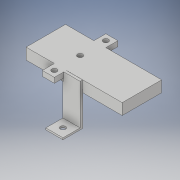
# Autodesk Inventor part: New poe ethernet splitter holder
Saved by Autodesk Inventor 2018 (Build 220112000, 112)
## iProperties
Created: 2019-11-08
Part Number: New poe ethernet splitter holder
Material: Generic
Document SubType Name: Modeling
Designer: Jacob
Density: 1 g/cm^3
Appearance: Default
Author: Jacob
Autodesk Inventor part; units mm, degrees
ref_plane "YZ Plane" through (0, 0, 0) normal (1, 0, 0) x (0, 1, 0)
ref_plane "XZ Plane" through (0, 0, 0) normal (0, 1, 0) x (-1, 0, 0)
ref_plane "XY Plane" through (0, 0, 0) normal (0, 0, 1) x (1, 0, 0)
sketch "Sketch1" plane through (0, 0, 0) normal (0, 1, 0) x (-1, 0, 0)
  line L0 (5, -5) -> (-5, -5)
  line L1 (-5, -5) -> (-5, 5)
  line L2 (-5, 5) -> (5, 5)
  line L3 (5, 5) -> (5, -5)
  line L4 (5, -5) -> (-5, 5) construction
  line L5 (-5, -5) -> (5, 5) construction
  circle A0 centre (0, 0) radius 1.5
  dimension "d0" = 10
  dimension "d1" = 10
  dimension "d2" = 3
  constraints: 12 end point, 2 midpoint, 2 parallel, 1 centre point, 1 coincident, 1 horizontal, 1 perpendicular
  measures "d0" distance of L0.start L0.end
  measures "d1" distance of L0.end L1.end
  measures "d2" diameter of A0
extrude "Extrusion1" add sketch "Sketch1" along normal blind 1
sketch "Sketch2" plane through (0, 1, 0) normal (0, 1, 0) x (1, 0, 0)
  line L0 (5, 5) -> (-5, 5) projected
  line L1 (-5, 5) -> (5, 5)
  line L2 (5, 5) -> (5, 6.5)
  line L3 (5, 6.5) -> (-5, 6.5)
  line L4 (-5, 6.5) -> (-5, 5)
  point P0 (0, 0)
  dimension "d5" = 1.5
  constraints: 8 end point, 2 parallel, 1 horizontal, 1 perpendicular
  measures "d5" distance of L1.end L2.end
extrude "Extrusion2" add sketch "Sketch2" against normal blind 1
sketch "Sketch3" plane through (0, 1, 0) normal (0, 1, 0) x (1, 0, 0)
  line L0 (-5, 6.5) -> (-5, -5) projected
  line L1 (5, -5) -> (5, 6.5) projected
  line L2 (-5, 6.5) -> (5, 6.5)
  line L3 (5, 6.5) -> (5, 5)
  line L4 (5, 5) -> (-5, 5)
  line L5 (-5, 5) -> (-5, 6.5)
  point P0 (0, 0)
  dimension "d8" = 1.5
  constraints: 8 end point, 2 parallel, 1 horizontal, 1 perpendicular, 1 point on line
  measures "d8" distance between parallel lines of L2 L4
extrude "Extrusion3" add sketch "Sketch3" along normal blind 17
sketch "Sketch4" plane through (0, 18, 0) normal (0, 1, 0) x (1, 0, 0)
  line L0 (-5, 5) -> (5, 5) projected
  line L1 (5, 6.5) -> (-5, 6.5) projected
  line L2 (-5, 6.5) -> (-5, 5) projected
  line L3 (5, 5) -> (5, 6.5) projected
  point P0 (0, 0)
extrude "Extrusion4" add sketch "Sketch4" along normal blind 1.5
sketch "Sketch5" plane through (5, 0, -6.5) normal (0, 0, -1) x (-1, 0, 0)
  line L0 (5, 0) -> (5, 19.5) construction
  line L1 (0, 19.5) -> (10, 19.5) projected
  line L2 (-23, 19.5) -> (33, 19.5)
  line L3 (33, 19.5) -> (33, 18)
  line L4 (33, 18) -> (-23, 18)
  line L5 (-23, 18) -> (-23, 19.5)
  line L6 (-23, 19.5) -> (33, 18) construction
  line L7 (33, 19.5) -> (-23, 18) construction
  point P0 (5, 18.75)
  dimension "d13" = 0
  dimension "d14" = 1.5
  dimension "d15" = 56
  constraints: 14 end point, 3 midpoint, 2 parallel, 1 horizontal, 1 perpendicular, 1 point on line
  measures "d13" distance between parallel lines of L1 L2
  measures "d14" distance of L4.end L2.start
  measures "d15" distance of L3.end L4.end
extrude "Extrusion5" add sketch "Sketch5" along normal blind 23
sketch "Sketch6" plane through (0, 19.5, 0) normal (0, 1, 0) x (1, 0, 0)
  line L0 (-28, 6.5) -> (-28, 29.5) projected
  line L1 (-28, 18) -> (28, 18) construction
  line L2 (28, 6.5) -> (28, 29.5) projected
  circle A0 centre (-8, 18) radius 1.5
  line L3 (-5, 6.5) -> (-28, 6.5) projected
  line L4 (-28, 29.5) -> (28, 29.5) projected
  line L5 (-5, 6.5) -> (5, 6.5) projected
  line L6 (28, 6.5) -> (5, 6.5) projected
  point P0 (0, 0)
  dimension "d18" = 20
  dimension "d19" = 3
  constraints: 2 end point, 2 midpoint, 1 centre point, 1 point on line
  measures "d18" distance from line of L0 A0.centre
  measures "d19" diameter of A0
extrude "Extrusion6" add sketch "Sketch6" along normal blind 5
sketch "Sketch8" plane through (0, 24.5, 0) normal (0, 1, 0) x (1, 0, 0)
  line L0 (-28, 6.5) -> (-28, 29.5) projected
  line L1 (-28, 18) -> (28, 18) construction
  line L2 (28, 6.5) -> (28, 29.5) projected
  line L3 (-28, 6.5) -> (-5, 6.5) projected
  line L4 (-8, 6.5) -> (-8, 29.5) construction
  line L5 (28, 29.5) -> (-28, 29.5) projected
  line L6 (-8, 18) -> (-8, 39.106) construction
  line L7 (-8, 18) -> (-8, -3.2826) construction
  line L8 (-11.5, 6.5) -> (-4.5, 6.5)
  line L9 (-4.5, 6.5) -> (-4.5, -0.5)
  line L10 (-4.5, -0.5) -> (-11.5, -0.5)
  line L11 (-11.5, -0.5) -> (-11.5, 6.5)
  line L12 (-11.5, 6.5) -> (-4.5, -0.5) construction
  line L13 (-4.5, 6.5) -> (-11.5, -0.5) construction
  line L14 (-11.5, 29.5) -> (-4.5, 29.5)
  line L15 (-4.5, 29.5) -> (-4.5, 36.5)
  line L16 (-4.5, 36.5) -> (-11.5, 36.5)
  line L17 (-11.5, 36.5) -> (-11.5, 29.5)
  line L18 (-11.5, 29.5) -> (-4.5, 36.5) construction
  line L19 (-4.5, 29.5) -> (-11.5, 36.5) construction
  circle A0 centre (-8, 3) radius 1.5
  circle A1 centre (-8, 33) radius 1.5
  point P0 (0, 0)
  dimension "d29" = 20
  dimension "d30" = 0
  dimension "d31" = 7
  dimension "d32" = 7
  dimension "d33" = 0
  dimension "d34" = 7
  dimension "d35" = 7
  dimension "d36" = 3
  dimension "d37" = 3
  constraints: 32 end point, 7 midpoint, 4 parallel, 4 point on line, 2 centre point, 2 coincident, 2 horizontal, 2 perpendicular, 2 vertical
  measures "d29" distance between parallel lines of L0 L4
  measures "d30" distance between parallel lines of L3 L8
  measures "d31" distance of L10.end L8.start
  measures "d32" distance of L9.end L10.end
  measures "d33" distance between parallel lines of L5 L14
  measures "d34" distance of L16.end L14.start
  measures "d35" distance of L15.end L16.end
  measures "d36" diameter of A0
  measures "d37" diameter of A1
extrude "Extrusion7" add sketch "Sketch8" against normal blind 3
sketch "Sketch9" plane through (0, 19.5, 0) normal (0, 1, 0) x (1, 0, 0)
  line L0 (5, 5) -> (5, 6.5) projected
  line L1 (-4.9196, 6.4645) -> (5, 6.4645)
  line L2 (5, 6.4645) -> (5, 5)
  line L3 (5, 5) -> (-4.9196, 5)
  line L4 (-4.9196, 5) -> (-4.9196, 6.4645)
  point P0 (0, 0)
  constraints: 8 end point, 2 parallel, 1 horizontal, 1 perpendicular
extrude "Extrusion8" add sketch "Sketch9" along normal blind 5
sketch "Sketch10" plane through (0, 24.5, 0) normal (0, 1, 0) x (1, 0, 0)
  circle A0 centre (-8, 18) radius 1.5 projected
  point P0 (0, 0)
extrude "Extrusion9" cut sketch "Sketch10" against normal blind 7
body "Solid1"
